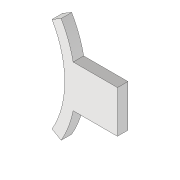
# Autodesk Inventor part: Finger
Saved by Autodesk Inventor 2020 (Build 240168000, 168)
## iProperties
Created: 2020-03-18
Part Number: Finger
Material: Generisch
Document SubType Name: Modeling
Designer: franz
Density: 1 g/cm^3
Appearance: Vorgabe
Author: franz
Autodesk Inventor part; units mm, degrees
ref_plane "YZ Plane" through (0, 0, 0) normal (1, 0, 0) x (0, 1, 0)
ref_plane "XZ Plane" through (0, 0, 0) normal (0, 1, 0) x (-1, 0, 0)
ref_plane "XY Plane" through (0, 0, 0) normal (0, 0, 1) x (1, 0, 0)
sketch "Skizze1" plane through (0, 0, 0) normal (1, 0, 0) x (0, 1, 0)
  line L0 (-10, -10) -> (-10, -5)
  line L1 (-10, -5) -> (-15, -5)
  line L2 (-15, -5) -> (-15, 0)
  line L3 (-15, 0) -> (15, 0)
  line L4 (15, 0) -> (15, -5)
  line L5 (15, -5) -> (10, -5)
  line L6 (10, -5) -> (10, -10)
  line L7 (10, -10) -> (20, -10)
  line L8 (20, -10) -> (20, -30)
  line L9 (20, -30) -> (-20, -30)
  line L10 (-20, -30) -> (-20, -10)
  line L11 (-20, -10) -> (-10, -10)
  line L12 (0, -36) -> (0, 6) projected
  point P0 (0, 0)
  dimension "d0" = 30
  dimension "d1" = 20
  dimension "d2" = 5
  dimension "d3" = 5
  dimension "d4" = 20
  dimension "d5" = 90
  dimension "d6" = 40
  constraints: 24 end point, 5 perpendicular, 2 parallel, 1 collinear, 1 midpoint, 1 point on line, 1 vertical, 5 other
  measures "d0" distance of L2.end L3.end
  measures "d1" distance between parallel lines of L6 L0
  measures "d2" distance of L1.end L2.end
  measures "d3" distance of L0.start L0.end
  measures "d4" distance between parallel lines of L11 L9
  measures "d5" angle of L7 L8
  measures "d6" distance of L7.end L10.end
extrude "Extrusion1" add sketch "Skizze1" along normal blind 10
sketch "Skizze3" plane through (0, 20, -10) normal (0, 1, 0) x (1, 0, 0)
  line L0 (0, 0) -> (0, 20) projected
  line L1 (0, 20) -> (40, 20)
  line L2 (40, 20) -> (40, 80)
  line L3 (40, 80) -> (-10, 80)
  line L4 (-10, 80) -> (-10, 90)
  line L5 (-10, 90) -> (50, 90)
  line L6 (50, 90) -> (50, 10)
  line L7 (50, 10) -> (0, 10)
  point P0 (0, -10)
  dimension "d12" = 10
  dimension "d13" = 10
  dimension "d14" = 10
  dimension "d15" = 60
  dimension "d16" = 50
  dimension "d17" = 60
  constraints: 14 end point, 6 perpendicular, 1 horizontal, 1 midpoint
  measures "d12" distance between parallel lines of L7 L1
  measures "d13" distance between parallel lines of L6 L2
  measures "d14" distance between parallel lines of L5 L3
  measures "d15" distance between parallel lines of L3 L1
  measures "d16" distance of L6.end L7.end
  measures "d17" distance of L4.end L5.end
extrude "Extrusion3" add sketch "Skizze3" against normal up to surface (40 mm away)
sketch "Skizze4" plane through (50, 20, -100) normal (0, 0, -1) x (-1, 0, 0)
  arc A0 (53.3975, 30) -> (53.3975, -70) centre (140, -20) ccw
  arc A1 (62.0577, 25) -> (62.0577, -65) centre (140, -20) ccw
  line L0 (140, -20) -> (53.3975, -70)
  line L1 (140, -20) -> (53.3975, 30)
  line L2 (0, -40) -> (60, -40) projected
  line L3 (0, 0) -> (60, 0) projected
  line L4 (0, 0) -> (0, -40) projected
  point P0 (40, -20)
  point P1 (42.0204, 0)
  point P2 (52.2504, 0)
  point P3 (52.2504, -40)
  point P4 (42.0204, -40)
  dimension "d20" = 200
  dimension "d21" = 180
  dimension "d22" = 30
  dimension "d23" = 30
  dimension "d24" = 40
  dimension "d25" = 20
  dimension "d30" = 140
  constraints: 5 point on circle, 4 end point, 2 centre point, 2 point on line, 1 coincident
  measures "d20" diameter of A0
  measures "d21" diameter of A1
  measures "d22" angle of L2 L0
  measures "d23" angle of L3 L1
  measures "d24" distance between parallel lines of L2 L3
  measures "d25" distance from line of L2 A0.centre
  measures "d30" distance from line of L4 A0.centre
extrude "Extrusion4" add sketch "Skizze4" against normal up to surface (10 mm away) contours L1 A1 L3 A0 | L2 A1 L0 A0
sketch "Skizze5" plane through (40, -20, -90) normal (0, 0, 1) x (1, 0, 0)
  arc A0 (-42.2504, 40) -> (-52.0577, 65) centre (-130, 20) ccw projected
  circle A1 centre (-130, 20) radius 90
  point P0 (-40, 20)
  point P1 (-52.0577, 65)
  point P2 (-42.2504, 40)
  constraints: 1 centre point, 1 coincident
extrude "Extrusion5" cut sketch "Skizze5" against normal up to surface (10 mm away)
sketch "Skizze6" plane through (40, -20, -90) normal (0, 0, 1) x (1, 0, 0)
  arc A0 (-52.0577, -25) -> (-52.0577, 65) centre (-130, 20) ccw projected
  line L0 (-43.3975, -30) -> (-52.0577, -25) projected
  arc A1 (-43.3975, -30) -> (-32.0204, 0) centre (-130, 20) ccw projected
  line L1 (-32.0204, 0) -> (0, 0) projected
  line L2 (0, 40) -> (0, 0) projected
  line L3 (-32.0204, 40) -> (0, 40) projected
  arc A2 (-32.0204, 40) -> (-43.3975, 70) centre (-130, 20) ccw projected
  line L4 (-52.0577, 65) -> (-43.3975, 70) projected
  line L5 (-30, 0) -> (-30, 40) projected
  line L6 (-30, 0) -> (10, 0) projected
  line L7 (10, 40) -> (10, 0) projected
  line L8 (-30, 40) -> (10, 40) projected
  point P0 (-40, 20)
extrude "Extrusion6" cut sketch "Skizze6" along normal through all
equation "\"d13\" = d12"
equation "\"d23\" = d22"
equation "\"d25\" = 0.5 * d24"
